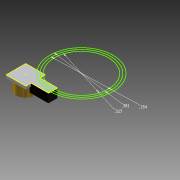
# Autodesk Inventor part: UMCC_Plug
Saved by Autodesk Inventor 2014 (Build 180170000, 170)
## iProperties
Created: 2015-11-06
Part Number: UMCC_Plug
Material: Generic
Document SubType Name: Modeling
Designer: Owner
Density: 1 g/cm^3
Appearance: Default
Author: Owner
Autodesk Inventor part; units mm, degrees
ref_plane "YZ Plane" through (0, 0, 0) normal (1, 0, 0) x (0, 1, 0)
ref_plane "XZ Plane" through (0, 0, 0) normal (0, 1, 0) x (-1, 0, 0)
ref_plane "XY Plane" through (0, 0, 0) normal (0, 0, 1) x (1, 0, 0)
sketch "Sketch1" plane through (0, 0, 0) normal (0, 1, 0) x (-1, 0, 0)
  line L0 (-1.5, 1.5) -> (1.5, 1.5)
  line L1 (1.5, 1.5) -> (1.5, -1.5)
  line L2 (1.5, -1.5) -> (-1.5, -1.5)
  line L3 (-1.5, -1.5) -> (-1.5, 1.5)
  point P0 (0, 0)
  dimension "d0" = 3
  dimension "d1" = 3
  dimension "d8" = 1.5
  dimension "d9" = 1.5
  constraints: 8 end point, 2 parallel, 1 horizontal, 1 perpendicular
  measures "d0" distance of L0.end L1.end
  measures "d1" distance of L0.start L0.end
  measures "d8" distance from line of L3 point (0, 0)
  measures "d9" distance from line of L2 point (0, 0)
extrude "Extrusion1" add sketch "Sketch1" along normal blind 0.5
sketch "Sketch2" plane through (0, 0, 0) normal (0, -1, 0) x (1, 0, 0)
  line L0 (1.5, -1.5) -> (1.5, 1.5) projected
  circle A0 centre (0, 0) radius 1.5
  circle A1 centre (0, 0) radius 1.399
  dimension "d4" = 2.7979
  dimension "d5" = 3
  constraints: 2 centre point, 1 coincident, 1 tangent
  measures "d4" diameter of A1
  measures "d5" diameter of A0
extrude "Extrusion2" add sketch "Sketch2" along normal blind 1.5
sketch "Sketch3" plane through (0, 0, 0) normal (0, 0, 1) x (1, 0, 0)
  line L0 (0, 0.5) -> (4.2, 0.5)
  line L1 (4.2, 0.5) -> (4.2, -0.87)
  line L2 (4.2, -0.87) -> (0, -0.87)
  line L3 (0, -0.87) -> (0, 0.5)
  line L4 (-1.5, 0) -> (-1.5, 0.5) projected
  line L5 (-1.5, 0.5) -> (1.5, 0.5) projected
  point P0 (0, 0)
  dimension "d10" = 5.7
  dimension "d11" = 1.37
  dimension "d12" = 0
  constraints: 8 end point, 2 parallel, 1 horizontal, 1 perpendicular
  measures "d10" distance between parallel lines of L1 L4
  measures "d11" distance of L0.end L1.end
  measures "d12" distance between parallel lines of L5 L0
extrude "Extrusion3" add sketch "Sketch3" along normal mid plane 1.37
sketch "Sketch4" plane through (0, 0.5, 0) normal (0, 1, 0) x (1, 0, 0)
  line L0 (1.5, 0.685) -> (1.5, 1.5) projected
  line L1 (1.5, 1.5) -> (-1.5, 1.5) projected
  line L2 (-1.5, 1.5) -> (-1.5, -1.5) projected
  line L3 (-1.5, -1.5) -> (1.5, -1.5) projected
  line L4 (1.5, -1.5) -> (1.5, -0.685) projected
  line L5 (4.2, -0.685) -> (1.5, -0.685) projected
  line L6 (4.2, -0.685) -> (4.2, 0.685) projected
  line L7 (1.5, 0.685) -> (4.2, 0.685) projected
  circle A0 centre (4.0858, 4.4759) radius 4.5
  circle A1 centre (4.0858, 4.4759) radius 4.1575
  circle A2 centre (4.0858, 4.4759) radius 4.8425
  circle A3 centre (4.2, -4.5313) radius 4.5
  circle A4 centre (4.2, -4.5313) radius 4.1575
  circle A5 centre (4.2, -4.5313) radius 4.8425
  point P0 (0, 0)
  dimension "d15" = 9
  dimension "d16" = 9.685
  dimension "d17" = 8.315
  dimension "d18" = 9
  dimension "d19" = 9.685
  dimension "d20" = 8.315
  constraints: 6 centre point, 4 coincident
  measures "d15" diameter of A0
  measures "d16" diameter of A2
  measures "d17" diameter of A1
  measures "d18" diameter of A3
  measures "d19" diameter of A5
  measures "d20" diameter of A4
body "Solid1"
